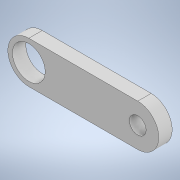
# Autodesk Inventor part: servo horn
Saved by Autodesk Inventor 2020 (Build 240168000, 168)
## iProperties
Created: 2026-07-08
Part Number: servo horn
Material: Generic
Document SubType Name: Modeling
Designer: drago
Density: 1 g/cm^3
Appearance: Default
Author: drago
Autodesk Inventor part; units mm, degrees
ref_plane "YZ Plane" through (0, 0, 0) normal (1, 0, 0) x (0, 1, 0)
ref_plane "XZ Plane" through (0, 0, 0) normal (0, 1, 0) x (-1, 0, 0)
ref_plane "XY Plane" through (0, 0, 0) normal (0, 0, 1) x (1, 0, 0)
sketch "Sketch1" plane through (0, 0, 0) normal (0, 0, 1) x (1, 0, 0)
  circle A0 centre (0, 0) radius 2.5
  circle A1 centre (13, 0) radius 1
  circle A2 centre (13, 0) radius 2.5
  line L0 (0, 2.5) -> (13, 2.5)
  line L1 (0, -2.5) -> (13, -2.5)
  circle A3 centre (0, 0) radius 1.9542
  dimension "d16" = 2
  dimension "d17" = 5
  constraints: 4 centre point, 4 end point, 4 point on circle, 2 coincident, 2 tangent
  measures "d16" diameter of A1
  measures "d17" diameter of A2
extrude "Extrusion1" add sketch "Sketch1" along normal blind 1.6
body "Solid1"
